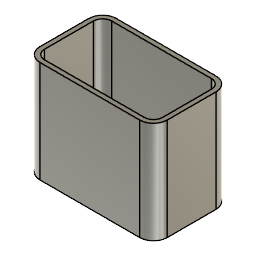
▢-125×75×4.5 (Autodesk Fusion 360 design; units mm, degrees)
Autodesk Fusion 360 part; units mm, degrees
sketch "スケッチ1" plane through (0, 0, 0) normal (0, 0, 1) x (1, 0, 0)
  arc A0 (449.3602, 239.3777) -> (462.8602, 252.8777) centre (449.3602, 252.8777) ccw
  arc A1 (449.3602, 243.8777) -> (458.3602, 252.8777) centre (449.3602, 252.8777) ccw
  arc A2 (337.8602, 252.8777) -> (351.3602, 239.3777) centre (351.3602, 252.8777) ccw
  arc A3 (342.3602, 252.8777) -> (351.3602, 243.8777) centre (351.3602, 252.8777) ccw
  line L0 (351.3602, 239.3777) -> (449.3602, 239.3777)
  line L1 (351.3602, 243.8777) -> (449.3602, 243.8777)
  line L2 (449.3602, 314.3777) -> (351.3602, 314.3777)
  line L3 (449.3602, 309.8777) -> (351.3602, 309.8777)
  line L4 (337.8602, 300.8777) -> (337.8602, 252.8777)
  line L5 (342.3602, 300.8777) -> (342.3602, 252.8777)
  arc A4 (351.3602, 314.3777) -> (337.8602, 300.8777) centre (351.3602, 300.8777) ccw
  arc A5 (351.3602, 309.8777) -> (342.3602, 300.8777) centre (351.3602, 300.8777) ccw
  line L6 (462.8602, 252.8777) -> (462.8602, 300.8777)
  line L7 (458.3602, 252.8777) -> (458.3602, 300.8777)
  arc A6 (462.8602, 300.8777) -> (449.3602, 314.3777) centre (449.3602, 300.8777) ccw
  arc A7 (458.3602, 300.8777) -> (449.3602, 309.8777) centre (449.3602, 300.8777) ccw
  point P0 (400.3602, 276.8777)
extrude "押し出し1" add sketch "スケッチ1" along normal blind 100
